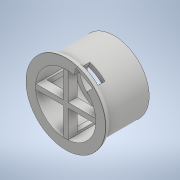
# Autodesk Inventor part: BaseRod_Pepu_2-01
Saved by Autodesk Inventor 2021 (Build 250183000, 183)
## iProperties
Created: 2020-11-14
Part Number: BaseRod_Pepu_2-01
Material: Genérico
Document SubType Name: Modeling
Designer: orgyn
Density: 1 g/cm^3
Appearance: Valor por defecto
Author: orgyn
Autodesk Inventor part; units mm, degrees
ref_plane "YZ Plane" through (0, 0, 0) normal (1, 0, 0) x (0, 1, 0)
ref_plane "XZ Plane" through (0, 0, 0) normal (0, 1, 0) x (-1, 0, 0)
ref_plane "XY Plane" through (0, 0, 0) normal (0, 0, 1) x (1, 0, 0)
sketch "Boceto1" plane through (0, 0, 0) normal (0, 1, 0) x (-1, 0, 0)
  circle A0 centre (0, 0) radius 62
  circle A1 centre (0, 0) radius 72
  circle A2 centre (0, 0) radius 52
  dimension "d5" = 124
  dimension "d6" = 144
  dimension "d7" = 104
  constraints: 3 centre point, 3 coincident
  measures "d5" diameter of A0
  measures "d6" diameter of A1
  measures "d7" diameter of A2
extrude "Extrusión1" add sketch "Boceto1" along normal blind 100 contours A1
sketch "Boceto5" plane through (0, 0, 0) normal (0, -1, 0) x (1, 0, 0)
  circle A0 centre (0, 0) radius 52
  circle A1 centre (0, 0) radius 62
  dimension "d11" = 104
  dimension "d12" = 124
  constraints: 2 centre point, 2 coincident
  measures "d11" diameter of A0
  measures "d12" diameter of A1
extrude "Extrusión2" add sketch "Boceto5" against normal blind 95
sketch "Boceto6" plane through (0, 0, 0) normal (0, -1, 0) x (1, 0, 0)
  circle A0 centre (0, 0) radius 52
  circle A1 centre (0, 0) radius 62
  dimension "d15" = 104
  dimension "d16" = 124
  constraints: 2 centre point, 2 coincident
  measures "d15" diameter of A0
  measures "d16" diameter of A1
extrude "Extrusión3" cut sketch "Boceto6" against normal blind 80
sketch "Boceto7" plane through (0, 0, 0) normal (0, -1, 0) x (1, 0, 0)
  circle A0 centre (0, 0) radius 82
  circle A1 centre (0, 0) radius 72
  dimension "d19" = 164
  dimension "d20" = 144
  constraints: 2 centre point, 2 coincident
  measures "d19" diameter of A0
  measures "d20" diameter of A1
extrude "Extrusión4" add sketch "Boceto7" against normal blind 15
fillet "Empalme1" radius 15 1 edges at (-82, 15, 0)
sketch "Boceto8" plane through (0, 0, 0) normal (0, -1, 0) x (1, 0, 0)
  arc A0 (43.8491, 43.8321) -> (16.8777, 59.6586) centre (0, 0) ccw
  line L0 (43.8491, 43.8321) -> (50.9216, 50.9018)
  line L1 (16.8777, 59.6586) -> (19.5999, 69.2809)
  line L2 (19.5999, 69.2809) -> (21.3442, 75.4464)
  line L3 (21.3442, 75.4464) -> (55.4532, 55.4317)
  line L4 (55.4532, 55.4317) -> (50.9216, 50.9018)
  dimension "d25" = 124
  constraints: 10 end point, 2 point on circle, 1 centre point
  measures "d25" diameter of A0
extrude "Extrusión5" cut sketch "Boceto8" against normal blind 30
sketch "Boceto9" plane through (0, 95, 0) normal (0, 1, 0) x (1, 0, 0)
  line L0 (51.775, -4.7614) -> (51.775, 6.1116)
  line L1 (5.2843, 55.289) -> (-4.7157, 55.289)
  line L2 (5.2843, 55.289) -> (5.2843, -56.0708)
  line L3 (5.2843, -56.0708) -> (-4.7157, -56.0708)
  line L4 (-4.7157, -56.0708) -> (-4.7157, 55.289)
  line L5 (5.2843, 55.289) -> (-4.7157, 55.289)
  line L6 (5.2843, 55.289) -> (5.2843, -56.0708)
  line L7 (5.2843, -56.0708) -> (-4.7157, -56.0708)
  line L8 (-4.7157, -56.0708) -> (-4.7157, 55.289)
  line L9 (-56.1571, 4.9777) -> (-56.1571, -5.0223)
  line L10 (-56.1571, 4.9777) -> (55.2027, 4.9777)
  line L11 (55.2027, 4.9777) -> (55.2027, -5.0223)
  line L12 (55.2027, -5.0223) -> (-56.1571, -5.0223)
  constraints: 26 end point, 6 perpendicular
extrude "Extrusión6" cut sketch "Boceto9" against normal blind 10
sketch "Boceto10" plane through (0, 85, 0) normal (0, 1, 0) x (1, 0, 0)
  line L0 (-51.7569, -5.0223) -> (-56.1571, -5.0223) projected
  line L1 (55.2027, -5.0223) -> (51.7569, -5.0223) projected
  line L2 (-56.1571, -5.0223) -> (55.2027, -5.0223)
  line L3 (55.2027, -5.0223) -> (55.2027, 4.9777)
  line L4 (-56.1571, 4.9777) -> (-51.7612, 4.9777) projected
  line L5 (55.2027, 4.9777) -> (-56.1571, 4.9777)
  line L6 (-56.1571, -5.0223) -> (-56.1571, 4.9777) projected
  line L7 (-56.1571, 4.9777) -> (-56.1571, -5.0223)
  line L8 (-4.7157, -56.0708) -> (-4.7157, -51.7857) projected
  line L9 (5.2843, -56.0708) -> (-4.7157, -56.0708) projected
  line L10 (-4.7157, -56.0708) -> (5.2843, -56.0708)
  line L11 (5.2843, 55.289) -> (5.2843, 51.7308) projected
  line L12 (5.2843, -56.0708) -> (5.2843, 55.289)
  line L13 (-4.7157, 55.289) -> (5.2843, 55.289) projected
  line L14 (5.2843, 55.289) -> (-4.7157, 55.289)
  line L15 (-4.7157, 55.289) -> (-4.7157, -56.0708)
  point P0 (0, 0)
  constraints: 16 end point, 5 perpendicular, 2 horizontal, 1 collinear
extrude "Extrusión7" add sketch "Boceto10" along normal blind 8
sketch "Boceto11" plane through (0, 85, 0) normal (0, -1, 0) x (1, 0, 0)
  circle A0 centre (0, 0) radius 67.1645
  line L0 (5.2843, 51.7308) -> (5.2843, 5.0223) projected
  line L1 (5.2843, 5.0223) -> (5.2843, 66.9563)
  line L2 (-4.7157, 5.0223) -> (-4.7157, 61.8204)
  circle A1 centre (0, 0) radius 62 projected
  line L3 (4.7157, 61.8204) -> (-4.7157, 61.8204)
  line L4 (-4.7157, 5.0223) -> (-61.7962, 5.0223)
  line L5 (-4.7496, -5.0223) -> (-61.7962, -5.0223)
  line L6 (-4.7157, -4.9777) -> (-51.7612, -4.9777) projected
  line L7 (-61.7962, 5.0223) -> (-61.7962, -5.0223)
  line L8 (-4.7157, -4.9777) -> (-4.7157, -61.8204)
  line L9 (51.7612, -4.9777) -> (5.2843, -4.9777) projected
  line L10 (5.2843, -4.9777) -> (5.2843, -61.8204)
  line L11 (5.2843, -61.8204) -> (-4.7157, -61.8204)
  line L12 (5.2843, -4.9777) -> (61.7999, -4.9777)
  line L13 (5.2843, 5.0223) -> (61.7962, 5.0223)
  line L14 (61.7999, -4.9777) -> (61.7962, 5.0223)
  line L15 (4.7157, 61.8204) -> (-4.7157, 61.8204)
  line L16 (-4.7157, -61.8204) -> (4.7157, -61.8204)
  line L17 (-61.7962, 5.0223) -> (-61.7962, -5.0223)
  line L18 (61.7962, -5.0223) -> (61.7962, 5.0223)
  line L19 (4.7157, -61.8204) -> (4.7157, -5.0223)
  line L20 (4.7157, 5.0223) -> (4.7157, 61.8204)
  line L21 (-4.7157, 61.8204) -> (-4.7157, 5.0223)
  line L22 (-4.7157, -4.9777) -> (-4.7157, -61.8204)
  line L23 (-61.7962, -5.0223) -> (-4.7157, -5.0223)
  line L24 (4.7157, -5.0223) -> (61.7962, -5.0223)
  line L25 (61.7962, 5.0223) -> (4.7157, 5.0223)
  line L26 (-4.7157, 5.0223) -> (-61.7962, 5.0223)
  constraints: 49 end point, 13 parallel, 8 perpendicular, 5 horizontal, 1 coincident, 1 collinear, 1 point on line, 1 vertical, 12 other
extrude "Extrusión8" add sketch "Boceto11" along normal blind 17.5 contours L13 L18 L12 L9 L10 L24 L19 L11 L8 L23 L5 L7 L4 L2 L3 L20 L25 | L3 A1 | L18 L24 L10 L9 L12
sketch "Boceto14" plane through (0, 93, 0) normal (0, 1, 0) x (1, 0, 0)
  line L0 (4.7157, 5.0223) -> (61.7962, 5.0223) projected
  line L1 (-51.7569, -5.0223) -> (-56.1571, -5.0223) projected
  line L2 (-56.1571, 5.0223) -> (-56.1571, -5.0223)
  line L3 (55.1889, -5.0223) -> (55.1889, 5.0223)
  line L4 (-4.7157, 55.289) -> (5.2843, 55.289) projected
  line L5 (-4.7157, -51.7857) -> (-4.7157, -61.8204) projected
  line L6 (5.2843, 55.289) -> (-4.7157, 55.289)
  line L7 (-4.7157, -56.1331) -> (5.2843, -56.1331)
  line L8 (5.2843, -56.1331) -> (5.2843, -5.0223)
  line L9 (5.2843, 5.0223) -> (5.2843, 55.289)
  line L10 (-56.1571, -5.0223) -> (-4.7157, -5.0223)
  line L11 (5.2843, -5.0223) -> (55.1889, -5.0223)
  line L12 (-4.7157, 55.289) -> (-4.7157, 5.0223)
  line L13 (-4.7157, -5.0223) -> (-4.7157, -56.1331)
  line L14 (55.1889, 5.0223) -> (5.2843, 5.0223)
  line L15 (-4.7157, 5.0223) -> (-56.1571, 5.0223)
  point P0 (0, 0)
  constraints: 24 end point, 10 parallel, 4 perpendicular, 3 horizontal, 2 point on line
extrude "Extrusión9" cut sketch "Boceto14" against normal blind 10
sketch "Boceto15" plane through (0, 67.5, 0) normal (0, -1, 0) x (1, 0, 0)
  line L0 (4.7157, 5.0223) -> (4.7157, 61.8204) projected
  line L1 (4.7157, 61.8204) -> (-4.7157, 61.8204)
  line L2 (-4.7157, -62.2061) -> (4.7157, -62.2061)
  line L3 (61.7962, 5.0223) -> (4.7157, 5.0223) projected
  line L4 (-68.0872, 5.0223) -> (-68.0872, -5.0019)
  line L5 (61.7962, -5.0019) -> (61.7962, 5.0223)
  line L6 (61.7962, 5.0223) -> (4.7157, 5.0223)
  line L7 (-4.7157, 5.0223) -> (-68.0872, 5.0223)
  line L8 (4.7157, -62.2061) -> (4.7157, -5.0019)
  line L9 (4.7157, 5.0223) -> (4.7157, 61.8204)
  line L10 (-68.0872, -5.0019) -> (-4.7157, -5.0019)
  line L11 (4.7157, -5.0019) -> (61.7962, -5.0019)
  line L12 (-4.7157, 61.8204) -> (-4.7157, 5.0223)
  line L13 (-4.7157, -5.0019) -> (-4.7157, -62.2061)
  point P0 (0, 0)
  constraints: 24 end point, 10 parallel, 4 perpendicular, 3 horizontal
extrude "Extrusión10" add sketch "Boceto15" along normal blind 67.25
sketch "Boceto16" plane through (0, 83, 0) normal (0, 1, 0) x (1, 0, 0)
  line L0 (-51.7569, -5.0223) -> (-56.1571, -5.0223) projected
  line L1 (-56.1571, 4.9777) -> (-56.1571, -5.0223)
  line L2 (5.2843, -56.1331) -> (-4.7157, -56.1331) projected
  line L3 (5.2843, 55.289) -> (5.2843, 51.7308) projected
  line L4 (-4.7157, -56.1331) -> (5.2843, -56.1331)
  line L5 (5.2843, 55.289) -> (-4.7157, 55.289)
  line L6 (56.7766, -5.86) -> (-57.5321, -5.86)
  line L7 (-57.5321, -5.86) -> (-57.5321, 5.884)
  line L8 (-57.5321, 5.884) -> (56.7766, 5.884)
  line L9 (56.7766, 5.884) -> (56.7766, -5.86)
  line L10 (7.1425, -57.6327) -> (-7.0826, -57.6327)
  line L11 (-7.0826, -57.6327) -> (-7.0826, 56.8297)
  line L12 (-7.0826, 56.8297) -> (7.1425, 56.8297)
  line L13 (7.1425, 56.8297) -> (7.1425, -57.6327)
  point P0 (55.2027, 4.9777)
  constraints: 22 end point, 5 parallel, 3 horizontal, 2 perpendicular
extrude "Extrusión11" cut sketch "Boceto16" against normal blind 64.5
